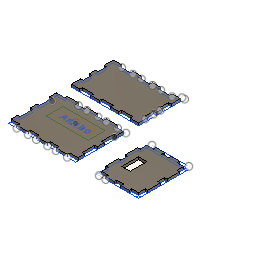
Plano_Caseta (v2~recovered) (Autodesk Fusion 360 design; units mm, degrees)
Autodesk Fusion 360 part; units mm, degrees
sketch "Sketch1" plane through (0, 0, 0) normal (0, 1, 0) x (1, 0, 0)
  line L0 (50, 50) -> (100, 50)
  line L1 (100, 50) -> (100, 30)
  line L2 (100, 30) -> (50, 30)
  line L3 (50, 30) -> (50, 50)
  line L4 (58.8512, 35.5366) -> (93.3385, 35.5366) construction
  line L5 (93.3385, 35.5366) -> (93.3385, 45.5366) construction
  line L6 (93.3385, 45.5366) -> (58.8512, 45.5366) construction
  line L7 (58.8512, 45.5366) -> (58.8512, 35.5366) construction
  line L8 (115, 60) -> (35, 60)
  line L9 (35, 60) -> (35, 0)
  line L10 (35, 0) -> (115, 0)
  line L11 (115, 0) -> (115, 60)
  line L12 (35, 60) -> (45, 60)
  line L13 (45, 60) -> (45, 57)
  line L14 (45, 57) -> (35, 57)
  line L15 (35, 57) -> (35, 60)
  line L16 (68.3333, 57) -> (58.3333, 57)
  line L17 (58.3333, 57) -> (58.3333, 60)
  line L18 (68.3333, 60) -> (68.3333, 57)
  line L19 (91.6667, 57) -> (81.6667, 57)
  line L20 (81.6667, 57) -> (81.6667, 60)
  line L21 (91.6667, 60) -> (91.6667, 57)
  line L22 (115, 57) -> (105, 57)
  line L23 (105, 57) -> (105, 60)
  line L24 (115, 60) -> (115, 57)
  line L25 (35, 75) -> (115, 75)
  line L26 (115, 75) -> (115, 125)
  line L27 (115, 125) -> (35, 125)
  line L28 (35, 125) -> (35, 75)
  line L29 (45, 3) -> (45, 0)
  line L30 (58.3333, 0) -> (58.3333, 3)
  line L31 (81.6667, 0) -> (81.6667, 3)
  line L32 (91.6667, 3) -> (91.6667, 0)
  line L33 (68.3333, 3) -> (68.3333, 0)
  line L34 (105, 0) -> (105, 3)
  line L35 (45, 3) -> (35, 3)
  line L36 (58.3333, 3) -> (68.3333, 3)
  line L37 (81.6667, 3) -> (91.6667, 3)
  line L38 (105, 3) -> (115, 3)
  line L39 (112, 49) -> (115, 49)
  line L40 (115, 49) -> (115, 34)
  line L41 (115, 34) -> (112, 34)
  line L42 (112, 34) -> (112, 49)
  line L43 (112, 26) -> (115, 26)
  line L44 (115, 26) -> (115, 11)
  line L45 (115, 11) -> (112, 11)
  line L46 (112, 11) -> (112, 26)
  line L47 (38, 49) -> (35, 49)
  line L48 (35, 49) -> (35, 34)
  line L49 (35, 34) -> (38, 34)
  line L50 (38, 34) -> (38, 49)
  line L51 (38, 26) -> (35, 26)
  line L52 (35, 26) -> (35, 11)
  line L53 (35, 11) -> (38, 11)
  line L54 (38, 11) -> (38, 26)
  line L55 (140, 60) -> (190, 60)
  line L56 (190, 60) -> (190, 0)
  line L57 (190, 0) -> (140, 0)
  line L58 (140, 0) -> (140, 60)
  line L59 (140, 57) -> (190, 57)
  line L60 (140, 3) -> (190, 3)
  line L61 (140, 49) -> (143, 49)
  line L62 (140, 34) -> (143, 34)
  line L63 (140, 26) -> (143, 26)
  line L64 (140, 11) -> (143, 11)
  line L65 (143, 49) -> (143, 60)
  line L66 (143, 26) -> (143, 34)
  line L67 (143, 11) -> (143, 0)
  line L68 (190, 49) -> (187, 49)
  line L69 (190, 34) -> (187, 34)
  line L70 (190, 26) -> (187, 26)
  line L71 (190, 11) -> (187, 11)
  line L72 (187, 49) -> (187, 60)
  line L73 (187, 34) -> (187, 26)
  line L74 (187, 11) -> (187, 0)
  line L75 (45, 75) -> (45, 78)
  line L76 (68.3333, 75) -> (68.3333, 78)
  line L77 (58.3333, 75) -> (58.3333, 78)
  line L78 (81.6667, 75) -> (81.6667, 78)
  line L79 (91.6667, 75) -> (91.6667, 78)
  line L80 (105, 75) -> (105, 78)
  line L81 (68.3333, 78) -> (81.6667, 78)
  line L82 (91.6667, 78) -> (105, 78)
  line L83 (58.3333, 78) -> (45, 78)
  line L84 (45, 122) -> (45, 125)
  line L85 (58.3333, 122) -> (58.3333, 125)
  line L86 (68.3333, 122) -> (68.3333, 125)
  line L87 (81.6667, 122) -> (81.6667, 125)
  line L88 (91.6667, 122) -> (91.6667, 125)
  line L89 (105, 122) -> (105, 125)
  line L90 (45, 122) -> (58.3333, 122)
  line L91 (68.3333, 122) -> (81.6667, 122)
  line L92 (91.6667, 122) -> (105, 122)
  line L93 (143, 63.0834) -> (151, 63.0834)
  line L94 (151, 63.0834) -> (161, 63.0834)
  line L95 (161, 63.0834) -> (169, 63.0834)
  line L96 (169, 63.0834) -> (179, 63.0834)
  line L97 (179, 63.0834) -> (187, 63.0834)
  line L98 (151, 60) -> (151, 57)
  line L99 (161, 60) -> (161, 57)
  line L100 (169, 60) -> (169, 57)
  line L101 (179, 60) -> (179, 57)
  line L102 (151, 3) -> (151, 0)
  line L103 (161, 3) -> (161, 0)
  line L104 (169, 3) -> (169, 0)
  line L105 (179, 3) -> (179, 0)
  line L106 (115, 129.9518) -> (112, 129.9518)
  line L107 (112, 125) -> (112, 75)
  line L108 (115, 114) -> (112, 114)
  line L109 (115, 104) -> (112, 104)
  line L110 (115, 96) -> (112, 96)
  line L111 (115, 86) -> (112, 86)
  line L112 (35, 114) -> (38, 114)
  line L113 (38, 114) -> (38, 104)
  line L114 (38, 104) -> (35, 104)
  line L115 (35, 96) -> (38, 96)
  line L116 (38, 96) -> (38, 86)
  line L117 (38, 86) -> (35, 86)
  point P0 (75, 40)
  point P1 (112, 49)
  point P2 (38, 49)
  dimension "d3" = 20
  dimension "d4" = 50
  dimension "d21" = 80
  dimension "d22" = 50
  dimension "d26" = 0
  dimension "d27" = -57
  dimension "d31" = 15
  dimension "d42" = 10
  dimension "d43" = 60
  dimension "d44" = 50
  dimension "d61" = 0
  dimension "d62" = 47
  dimension "d66" = 8
  dimension "d67" = 10
  dimension "d68" = 8
  dimension "d69" = 10
  dimension "d70" = 8
  dimension "d75" = 3
  constraint horizontal L0
  constraint vertical L1
  constraint horizontal L2
  constraint vertical L3
  constraint perpendicular L4 L5
  constraint parallel L4 L6
  constraint parallel L5 L7
  constraint perpendicular L8 L9
  constraint parallel L8 L10
  constraint parallel L9 L11
  constraint horizontal L8
  constraint horizontal L12
  constraint vertical L13
  constraint horizontal L14
  constraint vertical L15
  constraint horizontal L25
  constraint vertical L26
  constraint horizontal L27
  constraint vertical L28
  constraint coincident L9 L35.end
  constraint perpendicular L9 L35
  constraint perpendicular L33 L36
  constraint perpendicular L32 L37
  constraint coincident L11 L38.end
  constraint perpendicular L11 L38
  constraint horizontal L39
  constraint vertical L40
  constraint horizontal L41
  constraint vertical L42
  constraint coincident P1 L39.start
  constraint horizontal L43
  constraint vertical L44
  constraint horizontal L45
  constraint vertical L46
  constraint horizontal L47
  constraint vertical L48
  constraint horizontal L49
  constraint vertical L50
  constraint coincident P2 L47.start
  constraint horizontal L51
  constraint vertical L52
  constraint horizontal L53
  constraint vertical L54
  constraint horizontal L55
  constraint vertical L56
  constraint horizontal L57
  constraint vertical L58
  constraint coincident L58 L59.start
  constraint coincident L56 L59.end
  constraint perpendicular L56 L59
  constraint coincident L58 L60.start
  constraint coincident L56 L60.end
  constraint perpendicular L56 L60
  constraint coincident L58 L61.start
  constraint perpendicular L58 L61
  constraint coincident L58 L62.start
  constraint perpendicular L58 L62
  constraint coincident L58 L63.start
  constraint perpendicular L58 L63
  constraint coincident L58 L64.start
  constraint perpendicular L58 L64
  constraint coincident L55 L65.end
  constraint perpendicular L55 L65
  constraint perpendicular L63 L66
  constraint perpendicular L64 L67
  constraint coincident L56 L68.start
  constraint perpendicular L56 L68
  constraint coincident L56 L69.start
  constraint perpendicular L56 L69
  constraint coincident L56 L70.start
  constraint perpendicular L56 L70
  constraint coincident L56 L71.start
  constraint perpendicular L56 L71
  constraint coincident L55 L72.end
  constraint perpendicular L55 L72
  constraint perpendicular L70 L73
  constraint coincident L57 L74.end
  constraint perpendicular L57 L74
  constraint coincident L25 L75.start
  constraint perpendicular L25 L75
  constraint coincident L25 L76.start
  constraint perpendicular L25 L76
  constraint coincident L25 L77.start
  constraint perpendicular L25 L77
  constraint coincident L25 L78.start
  constraint perpendicular L25 L78
  constraint coincident L25 L79.start
  constraint perpendicular L25 L79
  constraint coincident L25 L80.start
  constraint perpendicular L25 L80
  constraint perpendicular L78 L81
  constraint perpendicular L80 L82
  constraint perpendicular L77 L83
  constraint perpendicular L85 L90
  constraint perpendicular L65 L93
  constraint perpendicular L65 L94
  constraint parallel L94 L95
  constraint parallel L94 L96
  constraint parallel L94 L97
  constraint coincident L55 L98.start
  constraint coincident L59 L98.end
  constraint perpendicular L59 L98
  constraint coincident L55 L99.start
  constraint coincident L59 L99.end
  constraint perpendicular L59 L99
  constraint coincident L55 L100.start
  constraint coincident L59 L100.end
  constraint perpendicular L59 L100
  constraint coincident L55 L101.start
  constraint coincident L59 L101.end
  constraint perpendicular L59 L101
  constraint coincident L60 L102.start
  constraint perpendicular L60 L102
  constraint coincident L60 L103.start
  constraint coincident L57 L103.end
  constraint perpendicular L57 L103
  constraint coincident L60 L104.start
  constraint coincident L57 L104.end
  constraint perpendicular L57 L104
  constraint coincident L60 L105.start
  constraint coincident L57 L105.end
  constraint perpendicular L57 L105
  constraint perpendicular L26 L106
  constraint coincident L27 L107.start
  constraint coincident L25 L107.end
  constraint perpendicular L25 L107
  constraint coincident L26 L108.start
  constraint coincident L107 L108.end
  constraint perpendicular L26 L108
  constraint coincident L26 L109.start
  constraint perpendicular L26 L109
  constraint coincident L26 L110.start
  constraint perpendicular L26 L110
  constraint coincident L26 L111.start
  constraint perpendicular L26 L111
  constraint coincident L28 L112.start
  constraint perpendicular L28 L112
  constraint perpendicular L108 L113
  constraint coincident L28 L114.end
  constraint perpendicular L28 L114
  constraint coincident L28 L115.start
  constraint perpendicular L28 L115
  constraint perpendicular L115 L116
  constraint coincident L28 L117.end
  constraint perpendicular L28 L117
  measures "d3" distance of L0.start L2.end
  measures "d4" distance of L0.start L0.end
  measures "d21" distance of L25.start L25.end
  measures "d22" distance of L25.start L27.end
  measures "d31" distance of P1 L41.end
  measures "d42" distance of L22.start L22.end
  measures "d43" distance of L10 L12
  measures "d44" distance of L55.start L55.end
  measures "d66" distance of L93.start L93.end
  measures "d67" distance of L93.end L94.end
  measures "d68" distance of L94.end L95.end
  measures "d69" distance of L95.end L96.end
  measures "d70" distance of L96.end L97.end
  measures "d75" distance of L112.start L112.end
extrude "Extrude1" add sketch "Sketch1" along normal blind 3 contours L0 L1 L2 L3 | L8 L9 L10 L11 L13 L14 L16 L17 L18 L19 L20 L21 L22 L23 L29 L30 L31 L32 L33 L34 L35 L36 L37 L38 L39 L41 L42 L43 L45 L46 L47 L49 L50 L51 L53 L54 makes body 1
sketch "Sketch2" plane through (0, 0, 0) normal (0, 1, 0) x (1, 0, 0)
extrude "Extrude2" add sketch "Sketch1" along normal blind 3 separate body contours L25 L27 L28 L75 L76 L77 L78 L79 L80 L81 L82 L83 L84 L85 L86 L87 L88 L89 L90 L91 L92 L107 L112 L113 L114 L115 L116 L117 | L25 L26 L107 L111 | L26 L107 L109 L110 | L26 L27 L107 L108 makes body 2
extrude "Extrude3" add sketch "Sketch1" along normal blind 3 separate body contours L55 L59 L98 L99 | L56 L58 L59 L60 L61 L62 L63 L64 L65 L66 L67 L68 L69 L70 L71 L72 L73 L74 | L55 L59 L100 L101 | L57 L60 L102 L103 | L57 L60 L104 L105 makes body 3
copy_body "Body->Comp1" bodies 1 removing the originals makes body 4 in component "Tapa_Z"
copy_body "Body->Comp2" bodies 3 removing the originals makes body 5 in component "Tapa_X"
copy_body "Body->Comp3" bodies 2 removing the originals makes body 6 in component "Tapa_Y"
sketch "Sketch3" plane through (0, 3, 0) normal (0, 1, 0) x (-1, 0, 0)
  line L0 (-190, -26) -> (-187, -26)
  line L1 (-187, -26) -> (-187, -34)
  line L2 (-187, -34) -> (-190, -34)
  line L3 (-190, -34) -> (-190, -49)
  line L4 (-190, -49) -> (-187, -49)
  line L5 (-187, -49) -> (-187, -57)
  line L6 (-187, -57) -> (-179, -57)
  line L7 (-179, -57) -> (-179, -60)
  line L8 (-179, -60) -> (-169, -60)
  line L9 (-169, -60) -> (-169, -57)
  line L10 (-169, -57) -> (-161, -57)
  line L11 (-161, -57) -> (-161, -60)
  line L12 (-161, -60) -> (-151, -60)
  line L13 (-151, -60) -> (-151, -57)
  line L14 (-151, -57) -> (-143, -57)
  line L15 (-143, -57) -> (-143, -49)
  line L16 (-143, -49) -> (-140, -49)
  line L17 (-140, -49) -> (-140, -34)
  line L18 (-140, -34) -> (-143, -34)
  line L19 (-143, -34) -> (-143, -26)
  line L20 (-143, -26) -> (-140, -26)
  line L21 (-140, -26) -> (-140, -11)
  line L22 (-140, -11) -> (-143, -11)
  line L23 (-143, -11) -> (-143, -3)
  line L24 (-143, -3) -> (-151, -3)
  line L25 (-151, -3) -> (-151, 0)
  line L26 (-151, 0) -> (-161, 0)
  line L27 (-161, 0) -> (-161, -3)
  line L28 (-161, -3) -> (-169, -3)
  line L29 (-169, -3) -> (-169, 0)
  line L30 (-169, 0) -> (-179, 0)
  line L31 (-179, 0) -> (-179, -3)
  line L32 (-179, -3) -> (-187, -3)
  line L33 (-187, -3) -> (-187, -11)
  line L34 (-187, -11) -> (-190, -11)
  line L35 (-190, -11) -> (-190, -26)
  line L36 (-150, -40) -> (-160, -40)
  line L37 (-160, -40) -> (-160, -20)
  line L38 (-160, -20) -> (-150, -20)
  line L39 (-150, -20) -> (-150, -40)
  dimension "d82" = 20
  dimension "d83" = 10
  constraint horizontal L36
  constraint vertical L37
  constraint horizontal L38
  constraint vertical L39
  measures "d82" distance of L36.start L38.end
  measures "d83" distance of L36.start L36.end
extrude "Extrude1'" cut sketch "Sketch3" against normal blind 3 contours L36 L37 L38 L39 bodies 5 in component "Tapa_X"
component "Tapa_Z" placed x (1, 0, 0) y (0, 1, 0) z (0, 0, 1) at (0, 0, 0)
component "Tapa_X" placed x (1, 0, 0) y (0, 1, 0) z (0, 0, 1) at (0, 0, 0)
component "Tapa_Y" placed x (1, 0, 0) y (0, 1, 0) z (0, 0, 1) at (0, 0, 0)
named bodies: "Tapa_Z", "Tapa_Y", "Tapa_X"
